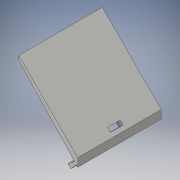
# Autodesk Inventor part: proto_1_panel
Saved by Autodesk Inventor 2016 (Build 200138000, 138)
## iProperties
Created: 2017-07-19
Part Number: proto_1_panel
Material: Generic
Document SubType Name: Modeling
Designer: Logan
Density: 1 g/cm^3
Appearance: Default
Author: Logan
Autodesk Inventor part; units mm, degrees
ref_plane "YZ Plane" through (0, 0, 0) normal (1, 0, 0) x (0, 1, 0)
ref_plane "XZ Plane" through (0, 0, 0) normal (0, 1, 0) x (-1, 0, 0)
ref_plane "XY Plane" through (0, 0, 0) normal (0, 0, 1) x (1, 0, 0)
sketch "Sketch1" plane through (0, 0, 0) normal (0, 0, 1) x (1, 0, 0)
  line L0 (-44.9013, 44.9013) -> (44.9013, -44.9013)
  line L1 (-44.9013, 44.9013) -> (82.0987, 44.9013) construction
  line L2 (-44.9013, 44.9013) -> (-44.9013, 38.5513)
  line L3 (44.9013, -44.9013) -> (44.9013, -57.6013)
  line L4 (44.9013, -57.6013) -> (-44.9013, 38.5513)
  line L5 (-44.9013, 38.5513) -> (-44.9013, -83.0013) construction
  line L6 (-44.9013, 38.5513) -> (76.6513, 38.5513) construction
  line L7 (44.9013, -57.6013) -> (80.8223, -57.6013) construction
  line L8 (44.9013, -57.6013) -> (37.9664, -50.1761) construction
  line L9 (37.9664, -50.1761) -> (84.3883, -50.1761) construction
  point P0 (0, 0)
  point P1 (0, 0)
  dimension "d0" = 127
  dimension "d1" = 45
  dimension "d2" = 6.35
  dimension "d5" = 12.7
  dimension "d6" = 90
  dimension "d10" = 10.16
  constraints: 20 end point, 4 horizontal, 2 equal length, 1 coincident, 1 midpoint, 1 perpendicular, 1 point on line, 1 vertical
  measures "d0" distance of L0.start L0.end
  measures "d1" angle of L0 L1
  measures "d2" distance of L0.start L2.end
  measures "d5" distance of L0.end L3.end
  measures "d6" angle of L5 L6
  measures "d10" distance of L3.end L8.end
extrude "Extrusion1" add sketch "Sketch1" against normal blind 127
sketch "Sketch4" plane through (37.9664, -50.1761, -101.6) normal (-0.7308, -0.6826, 0) x (0, 0, 1)
  line L0 (0, -1.5843) -> (0, 0) projected
  line L1 (101.6, 0) -> (101.6, -1.5843) projected
  line L2 (28.575, 11.43) -> (47.625, 11.43)
  line L3 (47.625, 11.43) -> (47.625, 5.08)
  line L4 (47.625, 5.08) -> (28.575, 5.08)
  line L5 (28.575, 5.08) -> (28.575, 11.43)
  line L6 (101.6, 0) -> (-25.4, 0) construction
  line L7 (-25.4, 126.0475) -> (-25.4, -0.8785) projected
  point P0 (101.6, 62.5845)
  point P1 (38.1, 5.08)
  point P2 (38.1, 0)
  dimension "d24" = 19.05
  dimension "d25" = 6.35
  dimension "d34" = 5.08
  constraints: 10 end point, 2 horizontal, 2 midpoint, 2 parallel, 1 perpendicular, 1 point on line, 1 vertical alignment
  measures "d24" distance of L3.end L4.end
  measures "d25" distance of L2.end L3.end
  measures "d34" distance of point (38.1, 0) point (38.1, 5.08)
extrude "Extrusion4" cut sketch "Sketch4" against normal up to next
sketch "Sketch5" plane through (0, 0, 0) normal (0, 0, 1) x (1, 0, 0)
  line L0 (44.9013, -57.6013) -> (37.9664, -50.1761) construction
  line L1 (44.9013, -57.6013) -> (-44.9013, 38.5513) projected
  line L2 (32.1524, -62.5572) -> (41.4339, -53.8887) construction
  line L3 (40.1336, -52.4965) -> (42.7341, -55.2809)
  line L4 (29.9852, -60.2368) -> (34.3195, -64.8776)
  line L5 (29.9852, -60.2368) -> (40.1336, -52.4965)
  line L6 (34.3195, -64.8776) -> (42.7341, -55.2809)
  point P0 (0, 0)
  dimension "d28" = 10.16
  dimension "d29" = 12.7
  dimension "d30" = 3.81
  dimension "d31" = 6.35
  constraints: 12 end point, 3 midpoint, 2 collinear, 1 parallel, 1 perpendicular
  measures "d28" distance of L0.start L0.end
  measures "d29" distance of L2.end L2.start
  measures "d30" distance of L3.start L3.end
  measures "d31" distance of L4.start L4.end
extrude "Extrusion5" add sketch "Sketch5" against normal blind 114.3
body "Solid1"
